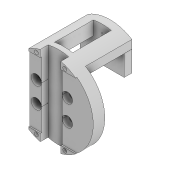
# Autodesk Inventor part: 55_spiralxy_slidemount_MGN7
Saved by Autodesk Inventor 2022 (Build 260153000, 153)
## iProperties
Created: 2023-09-18
Part Number: 55_spiralxy_slidemount_MGN7
Material: Generisch
Document SubType Name: Modeling
Designer: diederichbenedict
Density: 1 g/cm^3
Appearance: Vorgabe
Author: diederichbenedict
Autodesk Inventor part; units mm, degrees
ref_plane "YZ Plane" through (0, 0, 0) normal (1, 0, 0) x (0, 1, 0)
ref_plane "XZ Plane" through (0, 0, 0) normal (0, 1, 0) x (-1, 0, 0)
ref_plane "XY Plane" through (0, 0, 0) normal (0, 0, 1) x (1, 0, 0)
sketch "Skizze8" plane through (0, 0, 0) normal (0, 0, 1) x (1, 0, 0)
  line L0 (-8.5, -11.25) -> (8.5, -11.25)
  line L1 (8.5, -11.25) -> (8.5, 11.25)
  line L2 (8.5, 11.25) -> (-8.5, 11.25)
  line L3 (-8.5, 11.25) -> (-8.5, -11.25)
  line L4 (-8.5, -11.25) -> (8.5, 11.25) construction
  line L5 (8.5, -11.25) -> (-8.5, 11.25) construction
  line L6 (-8.5, 11.25) -> (8.5, 11.25)
  line L7 (8.5, 11.25) -> (8.5, 15.25)
  line L8 (8.5, 15.25) -> (-8.5, 15.25)
  line L9 (-8.5, 15.25) -> (-8.5, 11.25)
  line L10 (-6, -4) -> (6, -4) construction
  line L11 (6, -4) -> (6, 4) construction
  line L12 (6, 4) -> (-6, 4) construction
  line L13 (-6, 4) -> (-6, -4) construction
  line L14 (-6, -4) -> (6, 4) construction
  line L15 (6, -4) -> (-6, 4) construction
  circle A0 centre (-6, 4) radius 1
  circle A1 centre (6, 4) radius 1
  circle A2 centre (6, -4) radius 1
  circle A3 centre (-6, -4) radius 1
  circle A4 centre (0, 0) radius 15.2089
  line L16 (-8.5, -11.25) -> (-8.5, -12.6119)
  circle A5 centre (0, 0) radius 16
  line L17 (-8.5, -12.6119) -> (-8.5, -13.5554)
  point P0 (-8.5, 12.6119)
  point P1 (-8.5, 13.5554)
  dimension "d88" = 32
  dimension "d41" = 17
  dimension "d42" = 22.5
  dimension "d43" = 4
  dimension "d45" = 12
  dimension "d46" = 8
  dimension "d47" = 2
  dimension "d48" = 2
  dimension "d49" = 2
  dimension "d50" = 2
  constraints: 36 end point, 6 coincident, 6 parallel, 4 centre point, 4 midpoint, 3 horizontal, 3 perpendicular, 1 point on line, 1 vertical, 6 other
  measures "d41" distance of L2.end L1.end
  measures "d42" distance of L1.end L0.end
  measures "d43" distance of L7.end L6.end
  measures "d45" distance of L12.end L11.end
  measures "d46" distance of L11.end L10.end
  measures "d47" diameter of A0
  measures "d48" diameter of A1
  measures "d49" diameter of A2
  measures "d50" diameter of A3
extrude "Extrusion6" add sketch "Skizze8" along normal blind 5 contours L3 L2 L1 L0 | L0 L1 L7 A4 L16 | L9 A4 L7 L2 | A4 L7 A5 L17 | L9 A5 L8 L7 A4 | A5 L8
sketch "Skizze9" plane through (0, 0, 5) normal (0, 0, 1) x (1, 0, 0)
  circle A0 centre (-6, -4) radius 1 projected
  circle A1 centre (6, -4) radius 1 projected
  circle A2 centre (6, 4) radius 1 projected
  circle A3 centre (-6, 4) radius 1 projected
  point P0 (0, 0)
hole "Bohrung3" at (-6, -4, 5) at (6, -4, 5) at (6, 4, 5) at (-6, 4, 5) direction (0, 0, -1) diameter 2 depth 5 tip angle 118 counterbore diameter 4 counterbore depth 3
sketch "Skizze10" plane through (0, 0, 0) normal (0, 0, -1) x (-1, 0, 0)
  circle A0 centre (6, -4) radius 1 projected
  circle A1 centre (-6, -4) radius 1 projected
  circle A2 centre (-6, 4) radius 1 projected
  circle A3 centre (6, 4) radius 1 projected
  line L0 (-8.4771, 10.3023) -> (8.5, 10.3023)
  line L1 (-8.4771, 10.3023) -> (-8.4771, 12.6273)
  arc A4 (8.5, 13.5554) -> (8.5, -13.5554) centre (0, 0) ccw projected
  line L2 (8.5, 13.5554) -> (8.5, -13.5554) projected
  line L3 (8.5, 10.3023) -> (8.5, 13.5554)
  line L4 (-8.4771, 12.6273) -> (-8.4771, 13.5698)
  constraints: 8 end point, 2 vertical, 1 collinear, 1 horizontal, 1 point on circle
extrude "Extrusion7" add sketch "Skizze10" along normal blind 18 contours L1 L4 A4 L2 L0 picked at (0.6074, 12.1677)
sketch "Skizze11" plane through (0, 0, -18) normal (0, 0, -1) x (-1, 0, 0)
  line L0 (8.5, 10.3023) -> (-8.4771, 10.3023) projected
  line L1 (8.5, 10.3023) -> (8.5, -12.6119) projected
  line L2 (-8.5, 10.3364) -> (8.5, 10.3364)
  line L3 (8.5, 10.3364) -> (8.5, 2.3364)
  line L4 (8.5, 2.3364) -> (-8.5, 2.3364)
  line L5 (-8.5, 2.3364) -> (-8.5, 10.3364)
  line L6 (-8.4771, 10.3023) -> (8.5, 10.3023) projected
  line L7 (-8.4771, 13.5698) -> (-8.4771, 10.3023) projected
  line L8 (8.5, 10.3023) -> (8.5, 13.5554) projected
  arc A0 (8.5, 13.5554) -> (-8.4771, 13.5698) centre (0, 0) ccw projected
  point P0 (8.5, -11.25)
  dimension "d63" = 8
  constraints: 8 end point, 2 parallel, 1 horizontal, 1 perpendicular, 1 point on line, 1 other
  measures "d63" distance of L2.end L3.end
extrude "Extrusion8" add sketch "Skizze11" against normal blind 3 contours L1 L4 L5 L2 L7 L0 | L0 L7 L2 L3
sketch "Skizze12" plane through (0, 0, -18) normal (0, 0, -1) x (-1, 0, 0)
  line L0 (-8.5, 2.3364) -> (8.5, 2.3364) projected
  line L1 (8.5, 2.3364) -> (8.5, 13.5554) projected
  circle A0 centre (0, 3.9021) radius 0.25
  line L2 (-8.4771, 13.5698) -> (-8.4771, 10.3364) projected
  line L3 (-8.4771, 10.3364) -> (-8.5, 10.3364) projected
  line L4 (-8.5, 10.3364) -> (-8.5, 2.3364) projected
  arc A1 (8.5, 13.5554) -> (-8.4771, 13.5698) centre (0, 0) ccw projected
  dimension "d66" = 0.5
  constraints: 1 centre point
  measures "d66" diameter of A0
extrude "Extrusion9" cut sketch "Skizze12" against normal blind 3 contours A0
pattern_linear "Rechteckige Anordnung1" count 10 spacing 1 along (0, 1, 0) of "Extrusion9"
sketch "Skizze13" plane through (-8.5, 10.3023, 0) normal (0, -1, 0) x (1, 0, 0)
  line L0 (0, -15) -> (16.9771, -15) projected
  line L1 (16.9771, 0) -> (16.9771, -15) projected
  line L2 (0, 0) -> (16.9771, 0) projected
  line L3 (0, 0) -> (0, -15) projected
  line L4 (0, -15) -> (16.9771, -15) projected
  line L5 (5, 0) -> (12, 0)
  line L6 (12, 0) -> (12, -15)
  line L7 (12, -15) -> (5, -15)
  line L8 (5, -15) -> (5, 0)
  line L9 (5, 0) -> (12, -15) construction
  line L10 (12, 0) -> (5, -15) construction
  point P0 (8.5, 0)
  point P1 (8.749, -15)
  point P2 (8.5, -7.5)
  dimension "d72" = 7
  constraints: 12 end point, 2 midpoint, 2 parallel, 1 horizontal, 1 perpendicular, 1 point on line
  measures "d72" distance of L6.end L7.end
extrude "Extrusion10" cut sketch "Skizze13" against normal blind 10 contours L8 L2 L6 L0
sketch "Skizze14" plane through (0, 0, 5) normal (0, 0, 1) x (1, 0, 0)
  circle A0 centre (6, 4) radius 2 projected
  circle A1 centre (-6, -4) radius 2 projected
  circle A2 centre (6, -4) radius 2 projected
  circle A3 centre (-6, 4) radius 2 projected
  line L0 (-4, -22.1494) -> (4, -22.1494)
  line L1 (4, -22.1494) -> (4, 22.1494)
  line L2 (4, 22.1494) -> (-4, 22.1494)
  line L3 (-4, 22.1494) -> (-4, -22.1494)
  line L4 (-4, -22.1494) -> (4, 22.1494) construction
  line L5 (4, -22.1494) -> (-4, 22.1494) construction
  point P0 (0, 0)
  constraints: 12 end point, 2 midpoint, 2 parallel, 1 horizontal, 1 perpendicular
extrude "Extrusion11" cut sketch "Skizze14" against normal blind 3 contours L1 L0 L3 L2
sketch "Skizze15" plane through (0, 0, 5) normal (0, 0, 1) x (1, 0, 0)
  circle A0 centre (6, 4) radius 2 projected
  circle A1 centre (6, -4) radius 2 projected
  line L0 (12.5, -12.75) -> (-12.5, -12.75)
  line L1 (-12.5, -12.75) -> (-12.5, 12.75)
  line L2 (-12.5, 12.75) -> (12.5, 12.75)
  line L3 (12.5, 12.75) -> (12.5, -12.75)
  line L4 (12.5, -12.75) -> (-12.5, 12.75) construction
  line L5 (-12.5, -12.75) -> (12.5, 12.75) construction
  line L6 (5.5, -13.75) -> (-5.5, -13.75)
  line L7 (-5.5, -13.75) -> (-5.5, 13.75)
  line L8 (-5.5, 13.75) -> (5.5, 13.75)
  line L9 (5.5, 13.75) -> (5.5, -13.75)
  line L10 (5.5, -13.75) -> (-5.5, 13.75) construction
  line L11 (-5.5, -13.75) -> (5.5, 13.75) construction
  line L12 (4, 15.4919) -> (4, 4) projected
  line L13 (4, 4) -> (4, -4) projected
  line L14 (4, -4) -> (4, -15.4919) projected
  arc A2 (4, -15.4919) -> (4, 15.4919) centre (0, 0) ccw projected
  point P0 (5.5, 13.75)
  dimension "d77" = 25
  dimension "d78" = 25.5
  dimension "d79" = 11
  dimension "d80" = 27.5
  constraints: 24 end point, 4 midpoint, 4 parallel, 3 coincident, 2 horizontal, 2 horizontal alignment, 2 perpendicular, 1 point on line
  measures "d77" distance of L1.end L2.end
  measures "d78" distance of L0.end L1.end
  measures "d79" distance of L7.end L8.end
  measures "d80" distance of L6.end L7.end
hole "Bohrung4" at (-5.5, 13.75, 5) at (5.5, 13.75, 5) at (5.5, -13.75, 5) at (-5.5, -13.75, 5) direction (0, 0, -1) diameter 1.5 end through all
sketch "Skizze16" plane through (0, 0, 5) normal (0, 0, 1) x (1, 0, 0)
  circle A0 centre (5.5, -13.75) radius 0.75 projected
  circle A1 centre (5.5, 13.75) radius 0.75 projected
  line L0 (4, 15.4919) -> (4, 4) projected
  circle A2 centre (6, 4) radius 2 projected
  line L1 (4, 4) -> (4, -4) projected
  circle A3 centre (6, -4) radius 2 projected
  line L2 (4, -4) -> (4, -15.4919) projected
  arc A4 (4, -15.4919) -> (4, 15.4919) centre (0, 0) ccw projected
  line L3 (-23.9087, -12.7) -> (23.9087, -12.7)
  line L4 (23.9087, -12.7) -> (23.9087, 12.7)
  line L5 (23.9087, 12.7) -> (-23.9087, 12.7)
  line L6 (-23.9087, 12.7) -> (-23.9087, -12.7)
  line L7 (-23.9087, -12.7) -> (23.9087, 12.7) construction
  line L8 (23.9087, -12.7) -> (-23.9087, 12.7) construction
  dimension "d89" = 25.4
  constraints: 12 end point, 2 horizontal alignment, 2 midpoint, 2 parallel, 1 horizontal, 1 perpendicular
  measures "d89" distance of L4.end L3.end
extrude "Extrusion12" cut sketch "Skizze16" against normal blind 0.5 contours A2 | A3 | L5 A4 L3 L2 L1 L0 | L0 L1 L2 L3 L6 L5 | L5 L4 L3 A4
